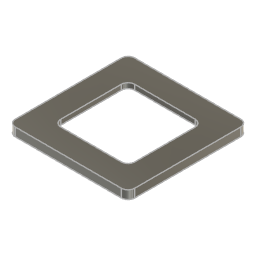
noita spell frame (Autodesk Fusion 360 design; units mm, degrees)
Autodesk Fusion 360 part; units mm, degrees
sketch "Sketch1" plane through (0, 0, 0) normal (0, 0, 1) x (1, 0, 0)
  line L0 (-9.7956, 28.3971) -> (18.7794, 28.3971)
  line L1 (21.9544, 25.2221) -> (21.9544, -3.3529)
  line L2 (18.7794, -6.5279) -> (-9.7956, -6.5279)
  line L3 (-12.9706, -3.3529) -> (-12.9706, 25.2221)
  line L4 (-20.5581, 39.1596) -> (29.5419, 39.1596)
  line L5 (32.7169, 35.9846) -> (32.7169, -14.1154)
  line L6 (29.5419, -17.2904) -> (-20.5581, -17.2904)
  line L7 (-23.7331, -14.1154) -> (-23.7331, 35.9846)
  arc A0 (-20.5581, 39.1596) -> (-23.7331, 35.9846) centre (-20.5581, 35.9846) ccw
  arc A1 (-9.7956, 28.3971) -> (-12.9706, 25.2221) centre (-9.7956, 25.2221) ccw
  arc A2 (21.9544, 25.2221) -> (18.7794, 28.3971) centre (18.7794, 25.2221) ccw
  arc A3 (32.7169, 35.9846) -> (29.5419, 39.1596) centre (29.5419, 35.9846) ccw
  arc A4 (29.5419, -17.2904) -> (32.7169, -14.1154) centre (29.5419, -14.1154) ccw
  arc A5 (18.7794, -6.5279) -> (21.9544, -3.3529) centre (18.7794, -3.3529) ccw
  arc A6 (-12.9706, -3.3529) -> (-9.7956, -6.5279) centre (-9.7956, -3.3529) ccw
  arc A7 (-23.7331, -14.1154) -> (-20.5581, -17.2904) centre (-20.5581, -14.1154) ccw
  circle A8 centre (26.4057, -10.9792) radius 3
  line L8 (21.9544, 10.9346) -> (-12.9706, 10.9346)
  line L9 (4.4919, -6.5279) -> (4.4919, 28.3971)
  circle A9 centre (4.4919, -11.9091) radius 3
  line L10 (21.0245, -5.5979) -> (24.2844, -8.8579) construction
  line L11 (21.0245, -5.5979) -> (21.383, -5.5979) construction
  line L12 (31.787, -16.3604) -> (28.527, -13.1005) construction
  line L13 (31.787, -16.3604) -> (27.9277, -16.3604) construction
  circle A10 centre (26.4057, 32.8484) radius 3
  circle A11 centre (27.3356, 10.9346) radius 3
  circle A12 centre (-17.4219, 32.8484) radius 3
  circle A13 centre (4.4919, 33.7784) radius 3
  circle A14 centre (-17.4219, -10.9792) radius 3
  circle A15 centre (-18.3519, 10.9346) radius 3
  line L14 (-14.5581, 29.9846) -> (23.5419, 29.9846)
  line L15 (23.5419, 29.9846) -> (23.5419, -8.1154)
  line L16 (23.5419, -8.1154) -> (-14.5581, -8.1154)
  line L17 (-14.5581, -8.1154) -> (-14.5581, 29.9846)
  line L18 (4.4919, 29.9846) -> (4.4919, -8.1154)
  line L19 (23.5419, 10.9346) -> (-14.5581, 10.9346)
  point P0 (-12.9706, 28.3971)
  point P1 (21.9544, 28.3971)
  point P2 (-12.9706, -6.5279)
  point P3 (4.4919, 10.9346)
  point P4 (4.4919, 10.9346)
  dimension "d1" = 34.925
  dimension "d2" = 34.925
  dimension "d3" = 10.7625
  dimension "d4" = 10.7625
  dimension "d5" = 10.7625
  dimension "d6" = 10.7625
  dimension "d7" = 3.175
  dimension "d8" = 6
  dimension "d11" = 6
  dimension "d16" = 45
  dimension "d17" = 135
  dimension "d18" = 5.3813
  dimension "d20" = 360
  dimension "d25" = 38.1
  dimension "d26" = 38.1
  constraint horizontal L0
  constraint vertical L1
  constraint horizontal L2
  constraint vertical L3
  constraint horizontal L4
  constraint vertical L5
  constraint horizontal L6
  constraint vertical L7
  constraint tangent L4 A0
  constraint tangent L7 A0
  constraint coincident P0 L0
  constraint coincident P0 L3
  constraint tangent L0 A1
  constraint tangent L3 A1
  constraint equal A0 A1
  constraint coincident P1 L0
  constraint coincident P1 L1
  constraint tangent L0 A2
  constraint tangent L1 A2
  constraint equal A0 A2
  constraint tangent L4 A3
  constraint tangent L5 A3
  constraint equal A0 A3
  constraint tangent L5 A4
  constraint tangent L6 A4
  constraint equal A0 A4
  constraint tangent L1 A5
  constraint tangent L2 A5
  constraint equal A0 A5
  constraint coincident P2 L2
  constraint coincident P2 L3
  constraint tangent L2 A6
  constraint tangent L3 A6
  constraint equal A0 A6
  constraint tangent L6 A7
  constraint tangent L7 A7
  constraint equal A0 A7
  constraint midpoint L1 L8.start
  constraint midpoint L3 L8.end
  constraint midpoint L2 L9.start
  constraint midpoint L0 L9.end
  constraint coincident L9 A9.centre
  constraint midpoint L8 P4
  constraint horizontal L11
  constraint midpoint A5 L10.start
  constraint coincident A8 L10.end
  constraint horizontal L13
  constraint midpoint A4 L12.start
  constraint coincident A8 L12.end
  constraint equal L10 L12
  constraint collinear A4.centre A5.centre A8.centre
  constraint horizontal L14
  constraint vertical L15
  constraint horizontal L16
  constraint vertical L17
  constraint midpoint L14 L18.start
  constraint midpoint L16 L18.end
  constraint midpoint L15 L19.start
  constraint midpoint L17 L19.end
  constraint midpoint L19 P4
  constraint coincident P4 P3
  measures "d1" distance of P0 P1
  measures "d2" distance of P0 P2
  measures "d3" distance of L0 L4
  measures "d4" distance of L3 L7
  measures "d5" distance of L2 L6
  measures "d6" distance of L1 L5
  measures "d7" radius of A0
  measures "d8" diameter of A8
  measures "d11" diameter of A9
  measures "d16" angle of L10 L11
  measures "d17" angle of L12 L13
  measures "d18" distance of L2 A9.centre
  measures "d25" distance of L14.start L14.end
  measures "d26" distance of L14.start L16.end
extrude "Extrude1" add sketch "Sketch1" along normal blind 2 contours L0 L3 A1 L14 L17 L18 L19 | L0 L1 A2 L14 L15 L18 L19 | L2 L3 A6 L16 L17 L18 L19 | L1 L2 A5 L15 L16 L18 L19 | L4 L5 L6 L7 A0 A3 A4 A7 | A8 | A9 | A10 | A11 | A12 | A13 | A14 | A15
extrude "Extrude2" add sketch "Sketch1" against normal blind 2 contours L0 L3 A1 L14 L17 L18 L19 | L0 L1 A2 L14 L15 L18 L19 | L2 L3 A6 L16 L17 L18 L19 | L1 L2 A5 L15 L16 L18 L19 | L4 L5 L6 L7 A0 A3 A4 A7
sketch "Sketch2" plane through (0, 0, -2) normal (0, 0, -1) x (1, 0, 0)
  circle A0 centre (27.3356, -10.9346) radius 3
  circle A1 centre (26.4057, 10.9792) radius 3
  circle A2 centre (26.4057, -32.8484) radius 3
  circle A3 centre (-17.4219, 10.9792) radius 3
  circle A4 centre (-17.4219, -32.8484) radius 3
  circle A5 centre (4.4919, -33.7784) radius 3
  circle A6 centre (4.4919, 11.9091) radius 3
  arc A7 (-12.9706, -25.2221) -> (-9.7956, -28.3971) centre (-9.7956, -25.2221) ccw
  line L0 (-12.9706, -25.2221) -> (-12.9706, 3.3529)
  arc A8 (-9.7956, 6.5279) -> (-12.9706, 3.3529) centre (-9.7956, 3.3529) ccw
  line L1 (-9.7956, 6.5279) -> (18.7794, 6.5279)
  arc A9 (21.9544, 3.3529) -> (18.7794, 6.5279) centre (18.7794, 3.3529) ccw
  line L2 (21.9544, 3.3529) -> (21.9544, -25.2221)
  arc A10 (18.7794, -28.3971) -> (21.9544, -25.2221) centre (18.7794, -25.2221) ccw
  line L3 (18.7794, -28.3971) -> (-9.7956, -28.3971)
  circle A11 centre (-18.3519, -10.9346) radius 3
  arc A12 (-23.7331, -35.9846) -> (-20.5581, -39.1596) centre (-20.5581, -35.9846) ccw
  line L4 (-20.5581, -39.1596) -> (29.5419, -39.1596)
  arc A13 (29.5419, -39.1596) -> (32.7169, -35.9846) centre (29.5419, -35.9846) ccw
  line L5 (32.7169, -35.9846) -> (32.7169, 14.1154)
  arc A14 (32.7169, 14.1154) -> (29.5419, 17.2904) centre (29.5419, 14.1154) ccw
  line L6 (29.5419, 17.2904) -> (-20.5581, 17.2904)
  arc A15 (-20.5581, 17.2904) -> (-23.7331, 14.1154) centre (-20.5581, 14.1154) ccw
  line L7 (-23.7331, 14.1154) -> (-23.7331, -35.9846)
  line L8 (23.5419, 8.1154) -> (-14.5581, 8.1154)
  line L9 (-14.5581, 8.1154) -> (-14.5581, -29.9846)
  line L10 (-14.5581, -29.9846) -> (23.5419, -29.9846)
  line L11 (23.5419, -29.9846) -> (23.5419, 8.1154)
extrude "Extrude3" cut sketch "Sketch2" against normal blind 1.5875 contours L8 L9 L10 L11
equation "d1 = d25 - 0.125 in"
equation "d2 = d1"
equation "d3 = d8 + 0.1875 in"
equation "d4 = d3"
equation "d5 = d3"
equation "d6 = d3"
equation "d11 = d8"
equation "d14 = d6 / 2"
equation "d18 = d5 / 2"
equation "d26 = d25"
